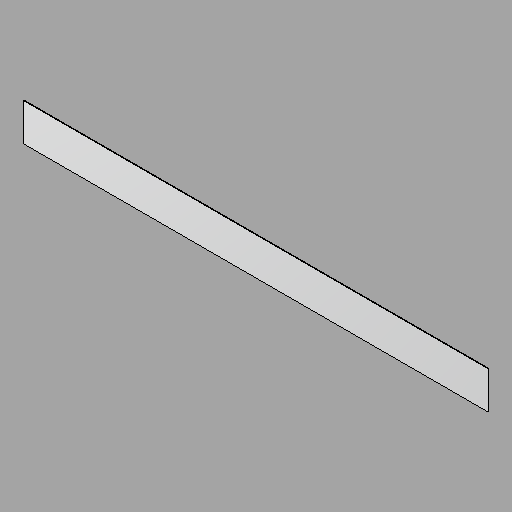
# Autodesk Inventor part: 板2
Saved by Autodesk Inventor 2022 (Build 260153000, 153)
## iProperties
Created: 2021-07-07
Part Number: 板2
Material: アルミニウム 6061
Document SubType Name: Modeling
Designer: nrz71
Density: 2.7 g/cm^3
Appearance: アルミニウム - フラット
Mass: 12.8732 g
Surface Area: 194.431 cm^2
Volume: 4.76784 cm^3
Author: nrz71
Autodesk Inventor part; units mm, degrees
ref_plane "YZ Plane" through (0, 0, 0) normal (1, 0, 0) x (0, 1, 0)
ref_plane "XZ Plane" through (0, 0, 0) normal (0, 1, 0) x (-1, 0, 0)
ref_plane "XY Plane" through (0, 0, 0) normal (0, 0, 1) x (1, 0, 0)
sketch "スケッチ1" plane through (0, 0, 0) normal (0, 0, 1) x (1, 0, 0)
  line L0 (-176, 2.5) -> (164, 2.5) projected
  line L1 (164, -25.22) -> (-176, -25.22) projected
  line L2 (-180, -105) -> (-180, 5) projected
  line L3 (164, -2.5) -> (164, 2.5) projected
  line L4 (-180, 2.5) -> (164, 2.5)
  line L5 (164, 2.5) -> (164, -25.22)
  line L6 (164, -25.22) -> (-180, -25.22)
  line L7 (-180, -25.22) -> (-180, 2.5)
  point P0 (0, 0)
  point P1 (-180, -25.22)
  constraints: 8 end point, 2 parallel, 1 horizontal, 1 perpendicular, 1 point on line
extrude "押し出し1" add sketch "スケッチ1" along normal blind 0.5
